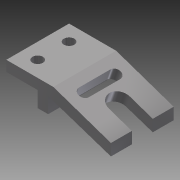
# Autodesk Inventor part: HW 7 Part 6
Saved by Autodesk Inventor 2015 (Build 190159000, 159)
## iProperties
Created: 2016-02-24
Part Number: HW 7 Part 6
Material: Steel, Mild
Document SubType Name: Modeling
Designer: Melissa
Density: 7.85 g/cm^3
Appearance: Semi-Polished
Mass: 983.163 g
Surface Area: 287.214 cm^2
Volume: 125.244 cm^3
Author: Melissa
Autodesk Inventor part; units mm, degrees
ref_plane "YZ Plane" through (0, 0, 0) normal (1, 0, 0) x (0, 1, 0)
ref_plane "XZ Plane" through (0, 0, 0) normal (0, 1, 0) x (-1, 0, 0)
ref_plane "XY Plane" through (0, 0, 0) normal (0, 0, 1) x (1, 0, 0)
sketch "Sketch1" plane through (0, 0, 0) normal (0, 0, 1) x (1, 0, 0)
  line L0 (0, 0) -> (12.7, 0)
  line L1 (12.7, 0) -> (12.7, 19.05)
  line L2 (12.7, 19.05) -> (88.9, -6.35)
  line L3 (88.9, -6.35) -> (88.9, 7.7874)
  line L4 (88.9, 7.7874) -> (19.05, 31.75)
  line L5 (19.05, 31.75) -> (-38.1, 31.75)
  line L6 (-38.1, 31.75) -> (-38.1, 19.05)
  line L7 (-38.1, 19.05) -> (0, 19.05)
  line L8 (0, 19.05) -> (0, 0)
  dimension "d9" = 38.1
  dimension "d10" = 12.7
  dimension "d11" = 19.05
  dimension "d12" = 38.1
  dimension "d13" = 12.7
  dimension "d14" = 127
  dimension "d15" = 57.15
  dimension "d16" = 0.5
  constraints: 18 end point, 3 parallel, 3 perpendicular, 1 horizontal, 1 vertical
  measures "d9" vertical distance of L2.end L5.end
  measures "d10" distance of L5.end L6.end
  measures "d11" vertical distance of L0.start L6.end
  measures "d12" distance of L6.end L7.end
  measures "d13" distance of L0.start L0.end
  measures "d14" horizontal distance of L2.end L6.end
  measures "d15" distance of L4.end L5.end
  measures "d16" angle of L2 L4
extrude "Extrusion1" add sketch "Sketch1" along normal mid plane 76.2
sketch "Sketch2" plane through (-38.1, 31.75, 38.1) normal (0, 1, 0) x (1, 0, 0)
  circle A0 centre (19.05, 19.05) radius 6.35
  circle A1 centre (19.05, 57.15) radius 6.35
  line L0 (57.15, 0) -> (0, 0) projected
  line L1 (0, 76.2) -> (0, 0) projected
  point P0 (38.1, 38.1)
  dimension "d19" = 12.7
  dimension "d20" = 12.7
  dimension "d21" = 0
  dimension "d22" = 38.1
  dimension "d23" = 19.05
  dimension "d24" = 19.05
  constraints: 2 centre point
  measures "d19" diameter of A0
  measures "d20" diameter of A1
  measures "d21" horizontal distance of A1.centre A0.centre
  measures "d22" distance of A1.centre A0.centre
  measures "d23" distance from line of A0.centre L0
  measures "d24" distance from line of L1 A0.centre
extrude "Extrusion2" cut sketch "Sketch2" against normal through all
sketch "Sketch3" plane through (19.05, 31.75, 38.1) normal (0.3244944, 0.9458876, 0) x (0.9458876, -0.3244944, 0)
  line L0 (19.05, 19.05) -> (19.05, 57.15) construction
  line L1 (12.7, 19.05) -> (12.7, 57.15)
  line L2 (25.4, 57.15) -> (25.4, 19.05)
  arc A0 (12.7, 19.05) -> (25.4, 19.05) centre (19.05, 19.05) ccw
  arc A1 (25.4, 57.15) -> (12.7, 57.15) centre (19.05, 57.15) ccw
  line L3 (-1.8853, 0) -> (78.4335, 0) projected
  line L4 (0, 76.2) -> (0, 0) projected
  line L5 (44.45, 25.4) -> (78.4335, 25.4)
  line L6 (78.4335, 76.2) -> (78.4335, 0) projected
  line L7 (78.4335, 50.8) -> (44.45, 50.8)
  arc A2 (44.45, 50.8) -> (44.45, 25.4) centre (44.45, 38.1) ccw
  point P0 (-7.7165, 38.1)
  point P1 (19.05, 38.1)
  dimension "d27" = 12.7
  dimension "d28" = 38.1
  dimension "d29" = 19.05
  dimension "d30" = 19.05
  dimension "d31" = 25.4
  dimension "d32" = 38.1
  dimension "d33" = 44.45
  constraints: 12 end point, 6 point on circle, 6 tangent, 3 centre point, 2 horizontal, 2 point on line, 1 midpoint, 1 parallel, 1 vertical
  measures "d27" distance between parallel lines of L2 L1
  measures "d28" distance of L0.end L0.start
  measures "d29" distance from line of L3 L0.start
  measures "d30" distance from line of L0.start L4
  measures "d31" distance between parallel lines of L7 L5
  measures "d32" vertical distance of L3.end A2.centre
  measures "d33" distance from line of L4 A2.centre
extrude "Extrusion3" cut sketch "Sketch3" against normal through all
body "Solid1"
